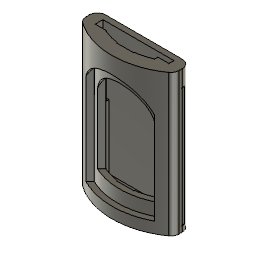
DIFFUSER(NEW) (Autodesk Fusion 360 design; units mm, degrees)
part number: 2026-03-04-21-54-54-099
Autodesk Fusion 360 part; units mm, degrees
sketch "BASE" plane through (0, 0, 0) normal (0, 0, 1) x (1, 0, 0)
  line L0 (-15.734917, 4.962551) -> (17.815083, 4.962551)
  line L1 (17.815083, 4.962551) -> (17.815083, -6.087449)
  line L2 (17.815083, -6.087449) -> (-15.734917, -6.087449)
  line L3 (-15.734917, -6.087449) -> (-15.734917, 4.962551)
  line L4 (-11.734917, 2.962551) -> (13.815083, 2.962551)
  line L5 (13.815083, 2.962551) -> (13.815083, 1.162551)
  line L6 (13.815083, 1.162551) -> (-11.734917, 1.162551)
  line L7 (-11.734917, 1.162551) -> (-11.734917, 2.962551)
  line L8 (1.040083, 1.162551) -> (1.040083, -3.837449)
  line L9 (-11.734917, 2.962551) -> (-15.734917, 2.962551)
  line L10 (-15.734917, 2.962551) -> (-16.265247, 2.432221)
  line L11 (-16.265247, 2.432221) -> (-17.679461, 1.018007)
  line L12 (13.815083, 2.962551) -> (17.815083, 2.962551)
  line L13 (17.815083, 2.962551) -> (18.345413, 2.432221)
  line L14 (18.345413, 2.432221) -> (19.759626, 1.018007)
  line L15 (18.345413, 2.432221) -> (20.345413, 2.432221) construction
  line L16 (1.040083, -3.837449) -> (1.040083, -4.587449)
  line L17 (1.040083, -4.587449) -> (1.040083, -6.587449)
  arc A0 (-15.734917, 2.962551) -> (17.815083, 2.962551) centre (1.040083, 20.253773) ccw
  arc A1 (-16.265247, 2.432221) -> (18.345413, 2.432221) centre (1.040083, 20.253478) ccw
  arc A2 (-17.679461, 1.018007) -> (19.759626, 1.018007) centre (1.040083, 20.252773) ccw
  line L18 (-15.734917, 2.962551) -> (-14.320704, 4.376764)
  line L19 (-15.734917, 2.962551) -> (-13.734917, 2.962551) construction
  line L20 (17.815083, 2.962551) -> (16.400869, 4.376764)
  line L21 (17.815083, 2.962551) -> (19.815083, 2.962551) construction
  line L22 (1.040083, -3.837449) -> (1.040083, -1.837449)
  arc A3 (-14.320704, 4.376764) -> (16.400869, 4.376764) centre (1.040083, 20.254663) ccw
  line L23 (1.040083, -1.837449) -> (4.040083, -1.837449)
  line L24 (1.040083, -1.837449) -> (-1.959917, -1.837449)
  line L25 (-1.959917, -1.837449) -> (-1.959917, 1.162551)
  line L26 (4.040083, -1.837449) -> (4.040083, 1.162551)
  line L27 (-11.734917, 1.162551) -> (-7.734917, 1.162551)
  line L28 (13.815083, 1.162551) -> (9.815083, 1.162551)
  line L29 (-11.734917, 1.162551) -> (-11.734917, -3.352246)
  line L30 (13.815083, 1.162551) -> (13.815083, -3.352246)
  line L31 (-7.734917, 1.162551) -> (-7.734917, -5.112497)
  line L32 (9.815083, 1.162551) -> (9.815083, -5.112497)
  line L33 (-7.734917, -0.019971) -> (-11.298312, -3.583366)
  line L34 (-7.734917, -0.019971) -> (-2.695516, -0.019971) construction
  line L35 (9.815083, -0.019971) -> (13.378478, -3.583366)
  dimension "d1" = 33.55
  dimension "d2" = 11.05
  dimension "d3" = 25.55
  dimension "d4" = 1.8
  dimension "d5" = 2
  dimension "d6" = 4
  dimension "d7" = 5
  dimension "d8" = 135
  dimension "d9" = 0.75
  dimension "d10" = 2
  dimension "d11" = 12.775
  dimension "d12" = 135
  dimension "d13" = 0.75
  dimension "d14" = 45
  dimension "d15" = 2
  dimension "d16" = 0.75
  dimension "d17" = 2
  dimension "d18" = 2
  dimension "d19" = 45
  dimension "d20" = 135
  dimension "d21" = 2
  dimension "d22" = 2
  dimension "d23" = 3
  dimension "d24" = 3
  dimension "d35" = 4
  dimension "d36" = 4
  dimension "d39" = 135
  dimension "d40" = 90
  constraint horizontal L0
  constraint vertical L1
  constraint horizontal L2
  constraint vertical L3
  constraint horizontal L4
  constraint vertical L5
  constraint horizontal L6
  constraint vertical L7
  constraint perpendicular L6 L8
  constraint perpendicular L3 L9
  constraint parallel L10 L11
  constraint perpendicular L1 L12
  constraint horizontal L15
  constraint parallel L8 L16
  constraint parallel L16 L17
  constraint horizontal L19
  constraint horizontal L21
  constraint parallel L8 L22
  constraint perpendicular L8 L23
  constraint tangent A3 L24
  constraint perpendicular L6 L25
  constraint perpendicular L6 L26
  constraint perpendicular L7 L27
  constraint perpendicular L5 L28
  constraint perpendicular L27 L29
  constraint perpendicular L6 L30
  constraint perpendicular L6 L31
  constraint perpendicular L28 L32
  constraint horizontal L34
  measures "d5" distance of L0 L4
  measures "d6" distance of L3 L7
  measures "d8" angle of L9 L10
  measures "d11" distance of L7 L8
  measures "d12" angle of L12 L13
  measures "d14" angle of L14 L15
  measures "d19" angle of L18 L19
  measures "d20" angle of L20 L21
  measures "d39" angle of L33 L34
  measures "d40" angle of L33 L35
extrude "Extrude1" add sketch "BASE" against normal blind 2 contours L0 L1 L3 L4 L9 L12 L18 L20 A3 | L3 A0 A1 L29 | L9 L18 A3 | L7 L9 A0 A3 L29 | L5 L12 A0 A3 L30 | L1 A0 A1 L30 | L12 L20 A3 | L3 A1 A2 L29 | L7 L9 A3 | L6 A0 A3 L27 L29 L33 | A0 A1 L29 L33 | L1 A1 A2 L30 | L5 L12 A3 | A0 A1 L30 L35 | L6 A0 A3 L28 L30 L35 | L2 L3 A2 | A1 A2 L29 L33 | L4 L5 L6 L7 A3 L27 L28 | L6 L7 A3 L27 | A0 L31 L33 | A0 A1 L31 L33 | L1 L2 A2 | A1 A2 L30 L35 | L5 L6 A3 L28 | A0 A1 L32 L35 | A0 L32 L35 | A1 A2 L31 L33 | L6 A3 L27 L31 | L8 A0 L22 A3 L24 L25 L31 | L16 A0 A1 L31 | L6 A3 L25 L31 | A1 A2 L32 L35 | L6 A3 L28 L32 | L16 A0 A1 L32 | L8 A0 L22 A3 L23 L26 L32 | L6 A3 L26 L32 | L2 L17 A1 A2 L31 | L2 L17 A2 | L6 L8 A3 L25 | A3 L24 L25 | L2 L17 A2 | L2 L17 A1 A2 L32 | A3 L23 L26 | L6 L8 A3 L26 picked at (-3.218251, 3.90536) picked at (-15.315389, 2.239827) picked at (-14.618176, 3.742457) picked at (-13.442127, 1.855246) picked at (15.522292, 1.855246) picked at (17.395555, 2.239827) picked at (16.698341, 3.742457) picked at (-12.663058, -1.248541) picked at (-12.062687, 2.714642) picked at (-11.181726, 0.717911) picked at (-11.464384, -0.626408) picked at (14.743223, -1.248541) picked at (14.142852, 2.714642) picked at (13.544549, -0.626408) picked at (13.261891, 0.717911) picked at (-14.436791, -3.432812) picked at (-11.099542, -2.178064) picked at (0.040083, 2.362551) picked at (-11.554084, 1.750528) picked at (-8.241933, -1.252182) picked at (-7.968269, -2.625959) picked at (16.516957, -3.432812) picked at (13.179708, -2.178064) picked at (13.634249, 1.750528) picked at (10.048434, -2.625959) picked at (10.322099, -1.252182) picked at (-10.414071, -3.275641) picked at (-8.000099, 0.495262) picked at (-6.160848, -2.003813) picked at (-6.785347, -2.755204) picked at (-5.185418, 0.531108) picked at (12.494237, -3.275641) picked at (10.080265, 0.495262) picked at (8.865513, -2.755204) picked at (8.241014, -2.003813) picked at (7.265584, 0.531108) picked at (-1.672879, -5.527558) picked at (0.463945, -6.402213) picked at (-0.627731, 0.192894) picked at (-1.627731, -1.738893) picked at (1.616221, -6.402213) picked at (3.753044, -5.527558) picked at (3.707897, -1.738893) picked at (2.707897, 0.192894)
extrude "Extrude2" add 1 faces at (1.040083, 1.112551, -2) along direction (0, 0, -1) blind 2
extrude "Extrude3" cut sketch "BASE" against normal blind 2 contours L3 A0 A1 L29 | L1 A0 A1 L30 | A0 A1 L29 L33 | A0 A1 L30 L35 | A0 A1 L31 L33 | A0 A1 L32 L35 | L16 A0 A1 L31 | L16 A0 A1 L32 picked at (-15.315389, 2.239827) picked at (17.395555, 2.239827) picked at (-11.464384, -0.626408) picked at (13.544549, -0.626408) picked at (-7.968269, -2.625959) picked at (10.048434, -2.625959) picked at (-6.785347, -2.755204) picked at (8.865513, -2.755204)
extrude "Extrude4" add sketch "BASE" along normal blind 47 contours L0 L1 L3 L4 L9 L12 L18 L20 A3 | L9 L18 A3 | L12 L20 A3 picked at (-3.218251, 3.90536) picked at (-14.618176, 3.742457) picked at (16.698341, 3.742457)
extrude "Extrude5" cut sketch "BASE" against normal blind 4 contours L2 L3 A2 | L1 L2 A2 picked at (-14.436791, -3.432812) picked at (16.516957, -3.432812)
extrude "Extrude6" add sketch "BASE" along normal blind 47 contours L7 L9 A0 A3 L29 | L5 L12 A0 A3 L30 | L7 L9 A3 | L5 L12 A3 picked at (-13.442127, 1.855246) picked at (15.522292, 1.855246) picked at (-12.062687, 2.714642) picked at (14.142852, 2.714642)
extrude "Extrude7" add sketch "BASE" along normal blind 25 contours L6 A0 A3 L27 L29 L33 | L6 A3 L27 L31 picked at (-11.181726, 0.717911) picked at (-8.000099, 0.495262)
extrude "Extrude8" add sketch "BASE" along normal blind 47 contours L3 A1 A2 L29 | L1 A1 A2 L30 | L6 A0 A3 L28 L30 L35 | A1 A2 L29 L33 | A1 A2 L30 L35 | L6 A3 L28 L32 picked at (-12.663058, -1.248541) picked at (14.743223, -1.248541) picked at (13.261891, 0.717911) picked at (-11.099542, -2.178064) picked at (13.179708, -2.178064) picked at (10.080265, 0.495262)
extrude "Extrude9" add sketch "BASE" along normal blind 4 contours A0 L31 L33 | A0 L32 L35 | L8 A0 L22 A3 L24 L25 L31 | L8 A0 L22 A3 L23 L26 L32 picked at (-8.241933, -1.252182) picked at (10.322099, -1.252182) picked at (-6.160848, -2.003813) picked at (8.241014, -2.003813)
sketch "Sketch2" plane through (0, 0, 25) normal (0, 0, 1) x (-1, 0, 0)
  line L0 (11.734917, -1.162551) -> (11.734917, 0.171367)
  arc A0 (11.734917, 0.171367) -> (9.246075, 1.531129) centre (-1.040083, -20.253773) ccw
  line L1 (9.246075, 1.531129) -> (7.734917, 0.019971)
  line L2 (7.734917, 0.019971) -> (7.734917, -1.162551)
  line L3 (7.734917, -1.162551) -> (11.734917, -1.162551)
extrude "Extrude10" add sketch "Sketch2" along normal blind 22 contours L0 A0 L1 L2 L3 picked at (10.131051, -0.556005)
sketch "Sketch3" plane through (0, 0, 47) normal (0, 0, 1) x (-1, 0, 0)
  line L0 (11.734917, -2.962551) -> (-13.815083, -2.962551)
  line L1 (-13.815083, -2.962551) -> (-13.815083, -1.162551)
  line L2 (-13.815083, -1.162551) -> (-9.815083, -1.162551)
  line L3 (-9.815083, -1.162551) -> (-9.815083, 0.019971)
  line L4 (-9.815083, 0.019971) -> (-11.32624, 1.531129)
  arc A0 (-11.32624, 1.531129) -> (-17.815083, -2.962551) centre (-1.040083, -20.253773) ccw
  line L5 (-17.815083, -2.962551) -> (-17.815083, -4.962551)
  line L6 (-17.815083, -4.962551) -> (15.734917, -4.962551)
  line L7 (15.734917, -4.962551) -> (15.734917, -2.962551)
  arc A1 (15.734917, -2.962551) -> (9.246075, 1.531129) centre (-1.040083, -20.253773) ccw
  line L8 (9.246075, 1.531129) -> (7.734917, 0.019971)
  line L9 (7.734917, 0.019971) -> (7.734917, -1.162551)
  line L10 (7.734917, -1.162551) -> (11.734917, -1.162551)
  line L11 (11.734917, -1.162551) -> (11.734917, -2.962551)
  line L12 (11.734917, -2.962551) -> (7.734917, -2.962551)
  line L13 (7.734917, -2.962551) -> (7.734917, -0.162551)
  line L14 (7.734917, -0.162551) -> (11.734917, -0.162551)
  line L15 (11.734917, -0.162551) -> (11.734917, -2.962551)
  dimension "d49" = 2.8
  constraint horizontal L12
  constraint vertical L13
  constraint horizontal L14
  constraint vertical L15
extrude "Extrude11" cut sketch "Sketch3" against normal blind 22 contours L9 L10 L13 L14 L15 picked at (9.068251, -0.495884)
sketch "UPFLAT" plane through (0, 2.962551, 0) normal (0, -1, 0) x (1, 0, 0)
  line L0 (13.815083, 0) -> (13.815083, 47)
  line L1 (13.815083, 47) -> (-11.734917, 47)
  line L2 (-11.734917, 47) -> (-11.734917, 0)
  line L3 (-11.734917, 0) -> (13.815083, 0)
  line L4 (-11.734917, 47) -> (13.815083, 47)
  line L5 (13.815083, 47) -> (13.815083, 0)
  line L6 (13.815083, 0) -> (-11.734917, 0)
  line L7 (-11.734917, 0) -> (-11.734917, 47)
  line L8 (-9.245917, 47) -> (11.326083, 47)
  line L9 (11.326083, 47) -> (11.326083, 37)
  line L10 (11.326083, 37) -> (-9.245917, 37)
  line L11 (-9.245917, 37) -> (-9.245917, 47)
  line L12 (-11.298417, 47) -> (13.378583, 47)
  line L13 (13.378583, 47) -> (13.378583, 41)
  line L14 (13.378583, 41) -> (-11.298417, 41)
  line L15 (-11.298417, 41) -> (-11.298417, 47)
  line L16 (1.040083, 47) -> (1.040083, 37)
  line L17 (1.040083, 47) -> (1.040083, 41)
  line L18 (-9.245917, 37) -> (-9.245917, 29)
  line L19 (11.326083, 37) -> (11.326083, 29)
  arc A0 (11.326083, 29) -> (-9.245917, 29) centre (1.040083, 26.387388) ccw
  line L20 (1.040083, 37) -> (4.040083, 37)
  line L21 (-11.298417, 41) -> (-11.298417, 33)
  line L22 (13.378583, 41) -> (13.378583, 33)
  arc A1 (13.378583, 33) -> (-11.298417, 33.103049) centre (1.016687, 27.449005) ccw
  line L23 (-11.298417, 33) -> (13.378583, 33)
  line L24 (-9.245917, 29) -> (11.326083, 29)
  dimension "d52" = 25.55
  dimension "d53" = 47
  dimension "d54" = 25.55
  dimension "d82" = 20.572
  dimension "d83" = 10
  dimension "d84" = 10
  dimension "d85" = 2.489
  dimension "d86" = 24.677
  dimension "d87" = 6
  dimension "d88" = 6
  dimension "d89" = 0.4365
  dimension "d98" = 10
  dimension "d99" = 12.3385
  dimension "d101" = 180
  dimension "d102" = 8
  dimension "d103" = 8
  dimension "d104" = 3
  dimension "d105" = 8
  dimension "d106" = 8
  constraint horizontal L4
  constraint vertical L5
  constraint horizontal L6
  constraint vertical L7
  constraint horizontal L8
  constraint vertical L9
  constraint horizontal L10
  constraint vertical L11
  constraint horizontal L12
  constraint vertical L13
  constraint horizontal L14
  constraint vertical L15
  constraint perpendicular L8 L16
  constraint perpendicular L10 L18
  constraint perpendicular L10 L19
  constraint perpendicular L16 L20
  constraint perpendicular L14 L21
  constraint perpendicular L14 L22
  measures "d54" distance of L2 L5
  measures "d84" distance of L8 L10
  measures "d85" distance of L7 L11
  measures "d88" distance of L4 L14
  measures "d89" distance of L7 L15
  measures "d99" distance of L15 L16
  measures "d101" angle of L17 L18
sketch "TOP" plane through (0, 0, 47) normal (0, 0, 1) x (-1, 0, 0)
  line L0 (7.734917, -0.162551) -> (11.734917, -0.162551)
  line L1 (11.734917, -0.162551) -> (11.734917, -2.962551)
  line L2 (11.734917, -2.962551) -> (-13.815083, -2.962551)
  line L3 (-13.815083, -2.962551) -> (-13.815083, -1.162551)
  line L4 (-13.815083, -1.162551) -> (-9.815083, -1.162551)
  line L5 (-9.815083, -1.162551) -> (-9.815083, 0.019971)
  line L6 (-9.815083, 0.019971) -> (-11.32624, 1.531129)
  arc A0 (-11.32624, 1.531129) -> (-17.815083, -2.962551) centre (-1.040083, -20.253773) ccw
  line L7 (-17.815083, -2.962551) -> (-17.815083, -4.962551)
  line L8 (-17.815083, -4.962551) -> (15.734917, -4.962551)
  line L9 (15.734917, -4.962551) -> (15.734917, -2.962551)
  arc A1 (15.734917, -2.962551) -> (9.246075, 1.531129) centre (-1.040083, -20.253773) ccw
  line L10 (9.246075, 1.531129) -> (7.734917, 0.019971)
  line L11 (7.734917, 0.019971) -> (7.734917, -0.162551)
  line L12 (15.734917, -4.962551) -> (-17.815083, -4.962551)
  line L13 (-17.815083, -4.962551) -> (-17.815083, 6.087449)
  line L14 (-17.815083, 6.087449) -> (15.734917, 6.087449)
  line L15 (15.734917, 6.087449) -> (15.734917, -4.962551)
  line L16 (11.734917, -2.962551) -> (-13.815083, -2.962551)
  line L17 (-13.815083, -2.962551) -> (-13.815083, -1.162551)
  line L18 (-13.815083, -1.162551) -> (11.734917, -1.162551)
  line L19 (11.734917, -1.162551) -> (11.734917, -2.962551)
  line L20 (-1.040083, -1.162551) -> (-1.040083, 3.837449)
  line L21 (11.734917, -2.962551) -> (15.734917, -2.962551)
  line L22 (15.734917, -2.962551) -> (17.679461, -1.018007)
  line L23 (15.734917, -2.962551) -> (16.265247, -2.432221)
  line L24 (15.734917, -2.962551) -> (14.984917, -2.962551) construction
  line L25 (15.734917, -2.962551) -> (14.320704, -4.376764)
  line L26 (15.734917, -2.962551) -> (17.734917, -2.962551) construction
  line L27 (-13.815083, -2.962551) -> (-17.815083, -2.962551)
  line L28 (-17.815083, -2.962551) -> (-19.759626, -1.018007)
  line L29 (-17.815083, -2.962551) -> (-18.345413, -2.432221)
  line L30 (-17.815083, -2.962551) -> (-16.400869, -4.376764)
  line L31 (-17.815083, -2.962551) -> (-15.815083, -2.962551) construction
  line L32 (-1.040083, 3.837449) -> (-1.040083, 1.837449)
  line L33 (-1.040083, 3.837449) -> (-1.040083, 6.587449)
  line L34 (-1.040083, 3.837449) -> (-1.040083, 4.587449)
  line L35 (-1.040083, 1.837449) -> (-1.040083, 3.837449)
  arc A2 (14.320704, -4.376764) -> (-16.400869, -4.376764) centre (-1.040083, -20.254663) ccw
  arc A3 (15.734917, -2.962551) -> (-17.815083, -2.962551) centre (-1.040083, -20.253773) ccw
  arc A4 (16.265247, -2.432221) -> (-18.345413, -2.432221) centre (-1.040083, -20.253478) ccw
  arc A5 (17.679461, -1.018007) -> (-19.759626, -1.018007) centre (-1.040083, -20.252773) ccw
  line L36 (-1.040083, 1.837449) -> (-4.040083, 1.837449)
  line L37 (-4.040083, 1.837449) -> (-4.040083, -1.162551)
  line L38 (-1.040083, 1.837449) -> (1.959917, 1.837449)
  line L39 (1.959917, 1.837449) -> (1.959917, -1.162551)
  line L40 (11.734917, -1.162551) -> (7.734917, -1.162551)
  line L41 (7.734917, -1.162551) -> (7.734917, 0.019971)
  line L42 (7.734917, 0.019971) -> (11.298312, 3.583366)
  line L43 (-9.815083, 0.019971) -> (-13.378478, 3.583366)
  dimension "d55" = 33.55
  dimension "d56" = 11.05
  dimension "d57" = 5
  dimension "d58" = 12.775
  dimension "d59" = 135
  dimension "d60" = 2.75
  dimension "d61" = 135
  dimension "d62" = 0.75
  dimension "d63" = 135
  dimension "d64" = 2
  dimension "d65" = 135
  dimension "d66" = 2.75
  dimension "d67" = 0.75
  dimension "d68" = 45
  dimension "d69" = 2
  dimension "d70" = 2
  dimension "d71" = 2.75
  dimension "d72" = 0.75
  dimension "d73" = 3
  dimension "d74" = 3
  dimension "d81" = 4
  constraint horizontal L12
  constraint vertical L13
  constraint horizontal L14
  constraint vertical L15
  constraint horizontal L16
  constraint vertical L17
  constraint horizontal L18
  constraint vertical L19
  constraint vertical L20
  constraint horizontal L24
  constraint horizontal L26
  constraint parallel L28 L29
  constraint horizontal L31
  constraint parallel L20 L32
  constraint parallel L32 L33
  constraint parallel L33 L34
  constraint perpendicular L35 L36
  constraint perpendicular L18 L37
  constraint perpendicular L32 L38
  constraint perpendicular L18 L39
  constraint perpendicular L1 L40
  constraint parallel L10 L42
  constraint perpendicular L42 L43
  measures "d58" distance of L17 L20
  measures "d59" angle of L21 L22
  measures "d61" angle of L23 L24
  measures "d63" angle of L25 L26
  measures "d65" angle of L27 L28
  measures "d68" angle of L30 L31
extrude "Extrude12" add sketch "TOP" against normal blind 9 contours L10 L20 L32 L35 A2 A3 L38 L39 L42 | L6 L20 L32 L35 A2 A3 L36 L37 L43 | L15 A4 A5 L42 | L14 L33 A4 A5 L42 | L14 L33 A4 A5 L43 | L14 L33 A5 | L14 L33 A5 | L13 A4 A5 L43 picked at (4.121342, 2.550484) picked at (-6.201507, 2.550484) picked at (13.374339, 0.766838) picked at (1.612346, 5.534653) picked at (-3.692512, 5.534653) picked at (-0.463945, 6.402213) picked at (-1.616221, 6.402213) picked at (-15.454505, 0.766838)
extrude "Extrude13" cut 1 faces at (-9.682452, -3.572381, 38) along direction (0, 0, 1) blind 3
extrude "Extrude14" add 1 faces at (1.040083, -2.504116, 38) along direction (0, 0, -1) blind 1
sketch "Sketch6" plane through (0, 0, 41) normal (0, 0, -1) x (1, 0, 0)
  line L0 (11.888516, 2.093405) -> (13.378478, 3.583366)
  arc A0 (13.378478, 3.583366) -> (-11.298312, 3.583366) centre (1.040083, -20.252773) ccw
  line L1 (-11.298312, 3.583366) -> (-9.80835, 2.093405)
  arc A1 (11.888516, 2.093405) -> (-9.80835, 2.093405) centre (1.040083, -20.253478) ccw
extrude "Extrude15" add sketch "TOP" against normal blind 6 contours A1 L15 A3 A4 L42 picked at (15.07027, -2.041538)
extrude "Extrude16" add sketch "TOP" against normal blind 6 contours A0 L13 A3 A4 L43 picked at (-17.150435, -2.041538)
extrude "Extrude17" add sketch "TOP" against normal blind 6 contours L33 L34 A3 A4 L42 | L33 L34 A3 A4 L43 picked at (4.319511, 3.445498) picked at (-6.399676, 3.445498)
extrude "Extrude18" add 1 faces at (1.040083, -2.504116, 37) along direction (0, 0, -1) blind 8
extrude "Extrude19" add sketch "Sketch6" along normal blind 8 contours L0 A0 L1 A1 picked at (-9.682452, 3.572381)
extrude "Extrude20" cut sketch "UPFLAT" along normal blind 20 contours L10 L16 A1 | L19 A1 L23 | L10 L16 L20 A1 | L10 L19 A0 L20 A1 L23 | L18 L21 A1 L23 | L10 L18 A0 A1 L23 | A0 L23 picked at (0.446728, 39.628559) picked at (12.500899, 33.381507) picked at (2.630726, 38.293522) picked at (10.664302, 34.081228) picked at (-10.419853, 33.444605) picked at (-8.584136, 34.099413) picked at (1.040083, 34.333333)
extrude "Extrude21" add 1 faces at (1.040083, -2.504116, 33) along direction (0, 0, 1) blind 14
extrude "Extrude22" add 2 faces at (12.885849, -2.335231, 33) (-10.805683, -2.335231, 33) along direction (0, 0, 1) blind 14
extrude "Extrude23" cut sketch "UPFLAT" along normal blind 20 contours A0 L23 | A0 L23 L24 picked at (1.040083, 34.333333) picked at (3.806968, 30.333333)
extrude "Extrude24" add 2 faces at (-8.742251, -0.462797, 29) (10.822416, -0.129464, 29) along direction (0, 0, 1) blind 6
fillet "Fillet1" radius 3 4 edges at (17.815083, -0.69948, 21.5) (17.815083, 4.962551, 21.5) (-15.734917, -0.69948, 21.5) (-15.734917, 4.962551, 21.5)
equation "d85 = ( ( 25.55 - 20.572 ) / 2 ) * 1 mm"
equation "d89 = ( ( 25.55 - 24.677 ) / 2 ) * 1 mm"
